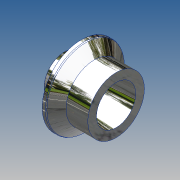
# Autodesk Inventor part: Propellernabe_ra8846s
Saved by Autodesk Inventor 2021 (Build 250183000, 183)
## iProperties
Created: 2020-11-16
Part Number: Propellernabe_ra8846s
Material: Aluminium 6061
Document SubType Name: Modeling
Designer: Ricardo A
Density: 2.7 g/cm^3
Appearance: Aluminium - flach
Description: Motor_teil6_nabe
Mass: 2.82642 g
Surface Area: 10.8874 cm^2
Volume: 1.04682 cm^3
Author: Sander
Revision Number: Rev00
Autodesk Inventor part; units mm, degrees
ref_plane "YZ-Ebene" through (0, 0, 0) normal (1, 0, 0) x (0, 1, 0)
ref_plane "XZ-Ebene" through (0, 0, 0) normal (0, 1, 0) x (-1, 0, 0)
ref_plane "XY-Ebene" through (0, 0, 0) normal (0, 0, 1) x (1, 0, 0)
sketch "Skizze1" plane through (0, 0, 0) normal (0, 0, 1) x (1, 0, 0)
  line L0 (-6.4, 0) -> (10.4, 0) projected
  line L1 (0, -1.8) -> (0, 10.8) projected
  line L2 (0, 9) -> (0.9023, 9)
  line L3 (0.9023, 9) -> (3, 6.5)
  line L4 (3, 6.5) -> (8, 6.5)
  line L5 (8, 6.5) -> (8, 4.5)
  line L6 (8, 4.5) -> (1.2, 3.82)
  line L7 (1.2, 3.82) -> (0, 3.7)
  line L8 (0, 3.7) -> (-4, 3.7)
  line L9 (-4, 3.7) -> (-4, 4.7)
  line L10 (-4, 4.7) -> (0, 5.85)
  line L11 (0, 5.85) -> (0, 9)
  point P0 (0, 0)
  dimension "d0" = 9
  dimension "d1" = 8
  dimension "d2" = 5
  dimension "d3" = 130
  dimension "d4" = 6.8
  dimension "d5" = 4
  dimension "d6" = 4.5
  dimension "d7" = 6.5
  dimension "d8" = 3.7
  dimension "d9" = 4.7
  dimension "d10" = 5.85
  constraints: 20 end point, 4 point on line, 2 horizontal, 2 perpendicular, 1 collinear, 1 parallel
  measures "d0" distance from line of L0 L2.start
  measures "d1" horizontal distance of L2.start L4.end
  measures "d2" distance of L3.end L4.end
  measures "d3" angle of L4 L3
  measures "d4" horizontal distance of L5.end L6.end
  measures "d5" distance of L7.end L8.end
  measures "d6" distance from line of L0 L5.end
  measures "d7" distance from line of L0 L4.end
  measures "d8" distance from line of L0 L8.end
  measures "d9" distance from line of L0 L9.end
  measures "d10" distance from line of L0 L10.end
revolve "Umdrehung1" add sketch "Skizze1" angle 360 about axis through (-10, 0, 0) along (1, 0, 0)
fillet "Rundung1" radius 0.3 3 edges at (0.9023, -9, 0) (-4, -4.7, 0) (-4, -3.7, 0)
